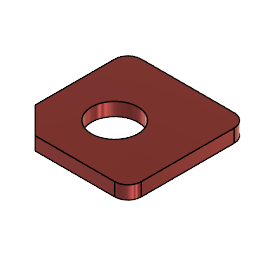
Baseplate (Autodesk Fusion 360 archive; units mm, degrees)
design "External1"
part number: 2026-01-26-22-02-14-008
Autodesk Fusion 360 part; units mm, degrees
other "DerivedContext1"
sketch "sketch 237" plane through (0, 0, 0) normal (0, 0, 1) x (1, 0, 0)
  line L0 (0, 0) -> (80, 0)
  line L1 (90, 10) -> (90, 80)
  line L2 (80, 90) -> (10, 90)
  line L3 (0, 80) -> (0, 0)
  line L4 (0, 20) -> (20, 0)
  circle A0 centre (40, 40) radius 17.5
  arc A1 (10, 90) -> (0, 80) centre (10, 80) ccw
  arc A2 (90, 80) -> (80, 90) centre (80, 80) ccw
  arc A3 (80, 0) -> (90, 10) centre (80, 10) ccw
  point P0 (90, 0)
  point P1 (0, 90)
extrude "Extrude1" add sketch "sketch 237" along normal blind 10 contours L0 L1 L2 L3 L4 A1 A2 A3
